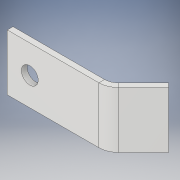
# Autodesk Inventor part: Piston Flag
Saved by Autodesk Inventor 2018 (Build 220112000, 112)
## iProperties
Created: 2017-09-25
Part Number: Piston Flag
Material: Nylon 6/6
Document SubType Name: Sheet Metal
Designer: Gabriel Smolnycki
Density: 1.13 g/cm^3
Sheet Metal Rule: 0.040 Al
Appearance: Smooth - White
Author: Gabriel Smolnycki
Autodesk Inventor part; units mm, degrees
note: some values were not read from the file. Chosen so that the rebuilt part matches the saved one: flange form of "Plate1".
ref_plane "YZ Plane" through (0, 0, 0) normal (1, 0, 0) x (0, 1, 0)
ref_plane "XZ Plane" through (0, 0, 0) normal (0, 1, 0) x (-1, 0, 0)
ref_plane "XY Plane" through (0, 0, 0) normal (0, 0, 1) x (1, 0, 0)
sketch "Sketch1" plane through (0, 0, 0) normal (0, 1, 0) x (-1, 0, 0)
  line L0 (0, 0) -> (-5.4801, -5.4801)
  line L1 (0, 0) -> (17.75, 0)
  dimension "d0" = 7.75
  dimension "d2" = 17.75
  dimension "d3" = 135
  measures "d0" distance of L0.start L0.end
  measures "d2" distance of L0.start L1.end
  measures "d3" angle of L0 L1
contour flange "Contour Flange1" sketch "Sketch1" thickness 1.016 bend radius 2.5 width 10 along (0, 1, 0) mid plane no both sides no wall seen from (2.74, 0, -2.74) lies toward (-0.7071068, 0, -0.7071068) curves L0 L1
bend "Bend1"
corner "Corner1"
sketch "Sketch2" plane through (-17.75, 0, -1.016) normal (0, 0, -1) x (-1, 0, 0)
  point P0 (-17.75, 0)
  point P1 (0, 0)
  point P2 (-4, 5)
  dimension "d15" = 5
  dimension "d16" = 4
  measures "d15" vertical distance of point (-4, 5) point (0, 0)
  measures "d16" horizontal distance of point (-4, 5) point (0, 0)
hole "Hole1" at (-13.75, 5, -1.016) direction (0, 0, 1) diameter 3 end through all
equation "\"d22\" = Thickness"
equation "\"d4\" = Thickness"
equation "\"d5\" = BendReliefWidth"
equation "\"d6\" = BendReliefDepth"
equation "\"d7\" = MinimumRemnant"
equation "\"d8\" = TransitionRadius"
equation "\"d12\" = CornerReliefSize"
equation "\"d13\" = GapSize"
equation "\"d14\" = JacobiRadiusSize"
equation "\"BendRadius\" = Thickness"
equation "\"BendReliefWidth\" = Thickness"
equation "\"BendReliefDepth\" = 0.5 * Thickness"
equation "\"CornerReliefSize\" = 4 * Thickness"
equation "\"MinimumRemnant\" = 2 * Thickness"
equation "\"TransitionRadius\" = BendRadius"
equation "\"JacobiRadiusSize\" = BendRadius"
equation "\"GapSize\" = Thickness"
equation "\"Thickness\" = 1.016"
body "Solid1"
